Autodesk Fusion 360 part; units mm, degrees
note: some values were not read from the file. Set by a fixed rule: which sketch regions a step uses.
(part 4 of 4)
  spline S146 degree 3 poles (26.5177, 7.8388) (26.6332, 7.8424) (26.7451, 7.8465) (26.8538, 7.8512) knots 0 0 0 0 0.059413 0.059413 0.059413 0.059413
  spline S147 degree 3 poles (26.8538, 7.8512) (26.956, 7.4679) (27.0677, 7.0952) (27.1887, 6.732) (27.7682, 4.9924) (28.5742, 3.4395) (29.7007, 2.1311) knots 0.438432 0.438432 0.438432 0.438432 0.510571 0.510571 0.510571 0.856047 0.856047 0.856047 0.856047
  spline S148 degree 3 poles (26.691, 29.369) (26.9094, 29.0796) (27.1485, 28.8139) (27.4084, 28.5686) (27.4895, 28.4921) (27.5725, 28.4177) (27.6573, 28.3455) (28.1077, 27.9624) (28.6062, 27.6405) (29.1383, 27.3828) knots 0.410269 0.410269 0.410269 0.410269 0.53135 0.53135 0.53135 0.569109 0.569109 0.569109 0.772757 0.772757 0.772757 0.772757
  spline S149 degree 3 poles (29.1383, 27.3828) (29.1539, 26.0141) (29.0974, 25.2619) (28.9645, 24.601) (28.94, 24.4789) (28.9124, 24.3583) (28.8809, 24.2344) (28.8291, 24.0307) (28.7663, 23.8183) (28.6865, 23.5786) knots 0.031454 0.031454 0.031454 0.031454 0.68068 0.68068 0.68068 0.800641 0.800641 0.800641 1 1 1 1
  spline S150 degree 3 poles (28.6865, 23.5786) (28.2125, 22.1565) (27.445, 21.3456) (26.7411, 20.9968) knots 0 0 0 0 1 1 1 1
  spline S151 degree 3 poles (26.7411, 20.9968) (26.3245, 20.7903) (26.1651, 20.7538) (26.0846, 20.7417) (26.0513, 20.7368) (26.0222, 20.7342) (25.9655, 20.7348) (25.9063, 20.7354) (25.8225, 20.7411) (25.6647, 20.7733) knots 0.000001 0.000001 0.000001 0.000001 0.502925 0.502925 0.502925 0.711303 0.711303 0.711303 1 1 1 1
  spline S152 degree 3 poles (25.6647, 20.7733) (24.9389, 20.9213) (24.3831, 21.2404) (23.8183, 21.9039) (23.6277, 22.1279) (23.4401, 22.3935) (23.2599, 22.7066) (22.8907, 23.3482) (22.5695, 24.1852) (22.3635, 25.2003) knots 0 0 0 0 0.489451 0.489451 0.489451 0.654705 0.654705 0.654705 1 1 1 1
  spline S153 degree 3 poles (22.3635, 25.2003) (22.2972, 25.5267) (22.198, 26.2499) (22.1289, 26.9737) (22.128, 26.983) (22.1271, 26.9923) (22.1263, 27.0016) knots 0 0 0 0 0.337072 0.337072 0.337072 0.341402 0.341402 0.341402 0.341402
  spline S154 degree 3 poles (22.1263, 27.0016) (22.211, 27.0082) (22.2987, 27.0165) (22.3856, 27.0265) (22.5004, 27.0396) (22.616, 27.056) (22.7315, 27.0758) (23.2642, 27.167) (23.6952, 27.3286) (24.0114, 27.4623) knots 0.424908 0.424908 0.424908 0.424908 0.500316 0.500316 0.500316 0.599835 0.599835 0.599835 1 1 1 1
  spline S155 degree 3 poles (24.0114, 27.4623) (24.9991, 27.8799) (25.9506, 28.4896) (26.691, 29.369) knots 0.000003 0.000003 0.000003 0.000003 0.49787 0.49787 0.49787 0.49787
  spline S156 degree 3 poles (44.1, 1.958) (46.0103, 3.7645) (47.4013, 6.008) (48.3961, 8.8894) (48.8667, 10.2525) (49.2674, 11.7642) (49.6499, 13.5042) knots 0 0 0 0 0.677783 0.677783 0.677783 1 1 1 1
  spline S157 degree 3 poles (49.6499, 13.5042) (50.6982, 18.2734) (51.1087, 21.6791) (51.3937, 27.8826) (51.3937, 27.8826) (51.3937, 27.8826) (51.3937, 27.8826) knots 0 0 0 0 1 1 1 1.000001 1.000001 1.000001 1.000001
  spline S158 degree 3 poles (51.417, 28.3722) (51.409, 28.2098) (51.4012, 28.0452) (51.3937, 27.8826) knots 1.469537 1.469537 1.469537 1.469537 1.67511 1.67511 1.67511 1.67511
  spline S159 degree 3 poles (51.417, 28.3722) (52.8091, 28.8275) (54.0786, 29.4972) (55.121, 30.4757) (55.2404, 30.5877) (55.3565, 30.7036) (55.469, 30.8234) (55.9481, 31.3332) (56.3598, 31.9144) (56.6765, 32.5579) knots 0.20705 0.20705 0.20705 0.20705 0.703865 0.703865 0.703865 0.760746 0.760746 0.760746 0.999997 0.999997 0.999997 0.999997
  spline S160 degree 3 poles (56.6765, 32.5579) (56.8802, 32.9718) (57.1032, 33.5033) (57.2076, 34.162) (57.2676, 34.5399) (57.2816, 34.8853) (57.2845, 35.1943) (57.2846, 35.1986) (57.2846, 35.2029) (57.2847, 35.2072) knots 0.000008 0.000008 0.000008 0.000008 0.549059 0.549059 0.549059 0.90483 0.90483 0.90483 0.910616 0.910616 0.910616 0.910616
  line L17 (57.2847, 35.2072) -> (57.2832, 35.6657)
  spline S161 degree 3 poles (57.2832, 35.6657) (57.2831, 35.6704) (57.283, 35.6751) (57.2829, 35.6798) (57.2757, 36.0979) (57.246, 36.5742) (57.1265, 37.0877) (57.0326, 37.4915) (56.904, 37.8404) (56.7766, 38.15) knots 0.082866 0.082866 0.082866 0.082866 0.088946 0.088946 0.088946 0.543269 0.543269 0.543269 0.908148 0.908148 0.908148 0.908148
  spline S162 degree 3 poles (56.7766, 38.15) (57.1856, 40.1641) (56.613, 42.1979) (55.3864, 43.7085) (55.3075, 43.8057) (55.2259, 43.9008) (55.1416, 43.9937) (54.1832, 45.05) (52.9102, 45.8137) (51.4736, 46.1975) knots 0.046261 0.046261 0.046261 0.046261 0.574454 0.574454 0.574454 0.608426 0.608426 0.608426 1 1 1 1
  spline S163 degree 3 poles (51.4736, 46.1975) (50.2108, 46.5348) (48.9151, 46.4935) (47.6271, 46.2315) knots 0.000001 0.000001 0.000001 0.000001 0.687909 0.687909 0.687909 0.687909
  spline S164 degree 3 poles (47.6271, 46.2315) (47.3607, 46.5511) (47.0576, 46.8619) (46.7108, 47.1487) (46.6375, 47.2093) (46.5591, 47.2712) (46.4754, 47.3329) knots 0.633034 0.633034 0.633034 0.633034 0.939053 0.939053 0.939053 0.999998 0.999998 0.999998 0.999998
  spline S165 degree 3 poles (46.4754, 47.3329) (45.0189, 48.4077) (43.2846, 48.7807) (41.6525, 48.7362) (41.0345, 48.7194) (40.4017, 48.6361) (39.771, 48.4665) knots 0.000002 0.000002 0.000002 0.000002 0.729882 0.729882 0.729882 1 1 1 1
  spline S166 degree 3 poles (39.771, 48.4665) (38.6073, 48.1535) (37.5427, 47.5875) (36.5857, 46.8757) knots 0.000002 0.000002 0.000002 0.000002 0.752898 0.752898 0.752898 0.752898
  spline S167 degree 3 poles (36.5857, 46.8757) (34.6398, 47.5736) (32.5086, 47.5041) (30.6605, 46.6256) (29.2239, 45.9427) (28.0213, 44.8138) (27.1748, 43.4008) knots 0.130761 0.130761 0.130761 0.130761 0.618328 0.618328 0.618328 1 1 1 1
  spline S168 degree 3 poles (27.1748, 43.4008) (26.7716, 42.7279) (26.4874, 41.9968) (26.3289, 41.2413) knots 0 0 0 0 0.28535 0.28535 0.28535 0.28535
  spline S169 degree 3 poles (26.3289, 41.2413) (25.7839, 42.057) (25.0421, 42.7849) (24.0925, 43.2821) (23.2389, 43.729) (22.3442, 43.9477) (21.4533, 44.0528) knots 0.123327 0.123327 0.123327 0.123327 0.510228 0.510228 0.510228 0.876075 0.876075 0.876075 0.876075
  spline S170 degree 3 poles (21.4533, 44.0528) (21.0452, 44.7091) (20.5419, 45.2814) (19.984, 45.7683) (19.3474, 46.3237) (18.5773, 46.8177) (17.6675, 47.124) knots 0.30885 0.30885 0.30885 0.30885 0.632884 0.632884 0.632884 1 1 1 1
  spline S171 degree 3 poles (17.6675, 47.124) (15.8473, 47.7367) (13.8817, 47.6408) (12.0388, 47.0023) (11.6314, 46.8612) (11.2289, 46.6965) (10.8282, 46.5111) knots 0 0 0 0 0.726997 0.726997 0.726997 0.890473 0.890473 0.890473 0.890473
  spline S172 degree 3 poles (10.8282, 46.5111) (9.9237, 47.1684) (8.9267, 47.6805) (7.8703, 48.0283) knots 3.010457 3.010457 3.010457 3.010457 3.200385 3.200385 3.200385 3.200385
  spline S173 degree 3 poles (7.8703, 48.0283) (6.7429, 48.3994) (5.5966, 48.5035) (4.5209, 48.4887) (3.7549, 48.4782) (2.9068, 48.4127) (2.0215, 48.1072) knots 0.000001 0.000001 0.000001 0.000001 0.579134 0.579134 0.579134 1 1 1 1
  spline S174 degree 3 poles (2.0215, 48.1072) (-0.6693, 47.1789) (-2.6359, 44.9494) (-3.079, 42.2803) (-3.2752, 41.0984) (-3.1629, 39.8642) (-2.7367, 38.7024) knots 0 0 0 0 0.618555 0.618555 0.618555 0.891277 0.891277 0.891277 0.891277
  spline S175 degree 3 poles (-2.7367, 38.7024) (-3.0358, 38.0066) (-3.2408, 37.2286) (-3.2572, 36.3894) (-3.2789, 35.282) (-2.9732, 34.2823) (-2.5712, 33.4233) knots 0.181215 0.181215 0.181215 0.181215 0.533212 0.533212 0.533212 1 1 1 1
  spline S176 degree 3 poles (-2.5712, 33.4233) (-1.6683, 31.4936) (-0.0223, 30.0814) (1.9142, 29.3886) knots 0 0 0 0 0.681546 0.681546 0.681546 0.681546
  spline S177 degree 3 poles (1.9142, 29.3886) (1.8905, 29.0144) (1.8662, 28.6344) (1.8438, 28.2882) knots 0.662826 0.662826 0.662826 0.662826 1 1 1 1
  spline S178 degree 3 poles (1.8438, 28.2882) (1.687, 25.8638) (1.7518, 22.7804) (2.0223, 20.5166) knots 0 0 0 0 1 1 1 1
  spline S179 degree 3 poles (2.0223, 20.5166) (2.6954, 14.8839) (4.9222, 9.8475) (8.5322, 5.9321) (8.9249, 5.5061) (9.3335, 5.0933) (9.7573, 4.6941) knots 2.814804 2.814804 2.814804 2.814804 3.207855 3.207855 3.207855 3.250613 3.250613 3.250613 3.250613
  spline S180 degree 3 poles (9.7573, 4.6941) (14.8102, -0.0653) (21.3375, -2.6228) (28.7072, -2.8617) (28.7072, -2.8617) (28.7072, -2.8617) (28.7072, -2.8617) knots 0 0 0 0 1 1 1 1.000001 1.000001 1.000001 1.000001
  spline S181 degree 3 poles (28.7072, -2.8617) (32.8949, -2.9973) (36.7147, -2.3353) (39.932, -0.8222) knots -0.538333 -0.538333 -0.538333 -0.538333 -0.206763 -0.206763 -0.206763 -0.206763
  spline S182 degree 3 poles (39.932, -0.8222) (41.5635, -0.0549) (42.8946, 0.8182) (44.1, 1.958) knots 0 0 0 0 1 1 1 1
  line L18 (42.9117, 54.5426) -> (42.9117, 52)
  line L19 (2.6189, 48.2805) -> (1.6128, 47.954)
  dimension "d26" = 2
  constraint vertical L18
  constraint coincident S173 L19.start
  constraint coincident S174 L19.end
hidden bodies 1 2
equation "CuttingHeight = 10 mm"
equation "IndentHeight = 5 mm"
equation "FlangeWidth = 2 mm"
equation "CutterWidth = 1.2 mm"
equation "d6 = -CutterWidth"
equation "FlangeThickness = 2 mm"
equation "d8 = -FlangeThickness"
equation "d10 = IndentHeight"
equation "d12 = CuttingHeight"
equation "d14 = -FlangeThickness"
equation "d16 = IndentHeight"
equation "d18 = CuttingHeight"
equation "d20 = FlangeThickness"
equation "d26 = FlangeWidth"
